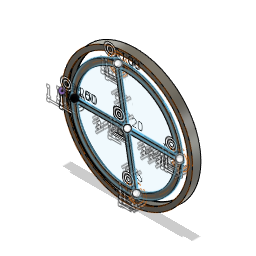
_Bottom ring 2.4a6c5033-3752-4bbe-af1c-aee209a3a47c (Autodesk Fusion 360 design; units mm, degrees)
Autodesk Fusion 360 part; units mm, degrees
sketch "Sketch1" plane through (0, 0, 0) normal (0, 1, 0) x (1, 0, 0)
  line L0 (0, 0) -> (0, 9)
  line L1 (0, 9) -> (1, 9)
  line L2 (0, 0) -> (1, 0)
  line L3 (1, 0) -> (4.84, 0)
  line L4 (4.84, 1.14) -> (2.2901, 3.3711)
  line L5 (2.2901, 5.6289) -> (5, 8)
  line L6 (5, 8) -> (5, 9)
  line L7 (5, 9) -> (1, 9)
  line L8 (4.84, 1.14) -> (4.84, 0)
  line L9 (0, 0) -> (4.84, 0)
  arc A0 (2.2901, 5.6289) -> (2.2901, 3.3711) centre (3.2779, 4.5) ccw
  line L10 (4.84, 0) -> (69.84, 0) construction
  line L11 (69.84, 0) -> (69.84, 13) construction
  dimension "d202" = 9
  dimension "d204" = 1.5
  dimension "d211" = 65
  constraint coincident L0.start L2.start
  constraint perpendicular L0 L1
  constraint perpendicular L3 L8
  constraint tangent L4 A0
  constraint tangent L5 A0
  constraint perpendicular L8 L10
  constraint perpendicular L10 L11
  measures "d202" distance of L0.start L0.end
  measures "d204" radius of A0
  measures "d211" distance of L3.end L10.end
revolve "Revolve2" add sketch "Sketch1" angle 360 about axis through (69.84, 0, 0) along (0, 0, -1) makes body 1
sketch "Sketch5" plane through (0, 0, 0) normal (0, 1, 0) x (1, 0, 0)
  line L0 (6.34, 8) -> (20.84, 8)
  line L1 (20.84, 1) -> (6.34, 1)
  arc A0 (20.84, 1) -> (20.84, 8) centre (20.84, 4.5) ccw
  arc A1 (6.34, 8) -> (6.34, 1) centre (6.34, 4.5) ccw
  line L2 (13.59, 8) -> (13.59, 1)
  line L3 (4.84, 0) -> (69.84, 0)
  line L4 (13.59, 1) -> (13.59, 0)
  dimension "d209" = 7
  dimension "d210" = 7
  constraint horizontal L0
  constraint horizontal L1
  constraint midpoint L0 L2.start
  constraint midpoint L1 L2.end
  constraint perpendicular L1 L2
  constraint coincident L3 L4.end
  constraint perpendicular L1 L4
  measures "d209" diameter of A1
  measures "d210" diameter of A0
sketch "Sketch6" plane through (0, 0, 0) normal (0, 0, 1) x (1, 0, 0)
  circle A0 centre (69.84, 0) radius 56.25 construction
  circle A1 centre (13.59, 0) radius 2.6
  circle A2 centre (13.59, 0) radius 8 construction
  circle A3 centre (13.59, 0) radius 10.75 construction
  circle A4 centre (69.84, 0) radius 69.84 construction
  circle A5 centre (69.84, 0) radius 65 construction
  circle A6 centre (60.0723, 55.3954) radius 10.75 construction
  circle A7 centre (60.0723, 55.3954) radius 8 construction
  circle A8 centre (60.0723, 55.3954) radius 2.6
  circle A9 centre (79.6077, -55.3954) radius 10.75 construction
  circle A10 centre (79.6077, -55.3954) radius 8 construction
  circle A11 centre (126.09, 0) radius 10.75 construction
  circle A12 centre (126.09, 0) radius 8 construction
  circle A13 centre (126.09, 0) radius 2.6
  circle A14 centre (79.6077, -55.3954) radius 2.6
  arc A15 (63.093, 58.8646) -> (56.0472, 57.6222) centre (60.0723, 55.3954) ccw
  arc A16 (122.9819, 3.3911) -> (63.9516, 52.9234) centre (69.84, 0) ccw
  arc A17 (128.9819, -3.5773) -> (128.9819, 3.5773) centre (126.09, 0) ccw
  arc A18 (128.9819, 3.5773) -> (63.093, 58.8646) centre (69.84, 0) ccw
  arc A19 (83.6328, -57.6222) -> (128.9819, -3.5773) centre (69.84, 0) ccw
  arc A20 (82.4076, -51.7457) -> (122.9819, -3.3911) centre (69.84, 0) ccw
  arc A21 (76.587, -58.8646) -> (83.6328, -57.6222) centre (79.6077, -55.3954) ccw
  arc A22 (57.2724, 51.7457) -> (16.6981, 3.3911) centre (69.84, 0) ccw
  arc A23 (16.6981, -3.3911) -> (75.7284, -52.9234) centre (69.84, 0) ccw
  arc A24 (56.0472, 57.6222) -> (10.6981, 3.5773) centre (69.84, 0) ccw
  arc A25 (10.6981, -3.5773) -> (76.587, -58.8646) centre (69.84, 0) ccw
  arc A26 (10.6981, 3.5773) -> (10.6981, -3.5773) centre (13.59, 0) ccw
  line L0 (17.7325, 2) -> (65.6975, 2)
  line L1 (17.7325, -2) -> (65.6975, -2)
  line L2 (71.0903, 4.4268) -> (62.7612, 51.6632)
  line L3 (62.0481, 55.7077) -> (62.0419, 55.7427)
  line L4 (67.1511, 3.7322) -> (58.822, 50.9686)
  line L5 (58.1089, 55.0131) -> (58.1027, 55.0481)
  arc A27 (57.2724, 51.7457) -> (58.822, 50.9686) centre (60.0723, 55.3954) ccw
  arc A28 (62.7612, 51.6632) -> (63.9516, 52.9234) centre (60.0723, 55.3954) ccw
  arc A29 (16.6981, -3.3911) -> (17.7325, -2) centre (13.59, 0) ccw
  arc A30 (17.7325, 2) -> (16.6981, 3.3911) centre (13.59, 0) ccw
  line L6 (81.5773, -55.0481) -> (81.5711, -55.0131)
  line L7 (80.858, -50.9686) -> (72.5289, -3.7322)
  line L8 (77.6381, -55.7427) -> (77.6319, -55.7077)
  line L9 (76.9188, -51.6632) -> (68.5897, -4.4268)
  arc A31 (82.4076, -51.7457) -> (80.858, -50.9686) centre (79.6077, -55.3954) ccw
  arc A32 (76.9188, -51.6632) -> (75.7284, -52.9234) centre (79.6077, -55.3954) ccw
  line L10 (73.9825, 2) -> (121.9475, 2)
  curve K0
  line L11 (73.9825, 2) -> (121.9475, 2)
  curve K1
  line L12 (73.9825, -2) -> (121.9475, -2)
  curve K2
  line L13 (73.9825, -2) -> (121.9475, -2)
  curve K3
  arc A33 (122.9819, 3.3911) -> (121.9475, 2) centre (126.09, 0) ccw
  arc A34 (121.9475, -2) -> (122.9819, -3.3911) centre (126.09, 0) ccw
  circle A35 centre (69.84, 0) radius 2.6
  arc A36 (65.6975, -2) -> (68.5897, -4.4268) centre (69.84, 0) ccw
  arc A37 (72.5289, -3.7322) -> (73.9825, -2) centre (69.84, 0) ccw
  arc A38 (73.9825, 2) -> (71.0903, 4.4268) centre (69.84, 0) ccw
  arc A39 (67.1511, 3.7322) -> (65.6975, 2) centre (69.84, 0) ccw
  circle A40 centre (69.84, 0) radius 3.6
  point P0 (13.59, 0)
  dimension "d213" = 5.2
  dimension "d214" = 16
  dimension "d215" = 21.5
  dimension "d219" = 5.2
  dimension "d220" = 16
  dimension "d221" = 21.5
  dimension "d224" = 5.2
  dimension "d225" = 5.2
  dimension "d236" = 5.2
  dimension "d238" = 1
  constraint coincident P0 A0
  constraint coincident P0 A1.centre
  constraint concentric A1 A3
  constraint coincident origin A4
  constraint concentric A6 A8
  constraint concentric A12 A13
  constraint concentric A9 A14
  constraint concentric A8 A27
  constraint concentric A15 A27
  constraint concentric A0 A22
  constraint concentric A0 A24
  constraint concentric A13 A33
  constraint coincident A17.end A24
  constraint coincident A16.start A22
  constraint concentric A16 A22
  constraint concentric A17 A33
  constraint concentric A18 A24
  constraint coincident A21.start A31
  constraint concentric A19 A24
  constraint concentric A20 A22
  constraint concentric A14 A31
  constraint concentric A21 A31
  constraint concentric A22 A23
  constraint coincident A24.end A29
  constraint concentric A24 A25
  constraint concentric A1 A29
  constraint concentric A26 A29
  constraint collinear L0 L10
  constraint collinear L1 L12
  constraint collinear L2 L6
  constraint collinear L4 L8
  constraint coincident A0 L3.start
  constraint collinear L2 L3
  constraint coincident A0 L5.start
  constraint collinear L4 L5
  constraint coincident L2.end A27
  constraint concentric A27 A28
  constraint coincident L0.start A29
  constraint concentric A29 A30
  constraint coincident A0 L6.end
  constraint collinear L6 L7
  constraint coincident A0 L8.end
  constraint collinear L8 L9
  constraint coincident L9.start A31
  constraint concentric A31 A32
  constraint coincident L12.end A33
  constraint concentric A33 A34
  constraint concentric A0 A35
  constraint coincident L10.start A37
  constraint coincident L2.start A37
  constraint coincident L4.start A37
  constraint coincident L1.end A37
  constraint concentric A35 A37
  constraint concentric A36 A37
  constraint concentric A37 A38
  constraint concentric A38 A39
  measures "d213" diameter of A1
  measures "d214" diameter of A2
  measures "d215" diameter of A3
  measures "d219" diameter of A8
  measures "d220" diameter of A7
  measures "d221" diameter of A6
  measures "d224" diameter of A13
  measures "d225" diameter of A14
  measures "d236" diameter of A35
extrude "Extrude36" add sketch "Sketch6" along normal blind 2 separate body contours A15 A17 A18 A19 A21 A24 A25 A26 makes body 2
extrude "Extrude37" add sketch "Sketch6" along normal blind 7.5 contours A40 bodies 2
